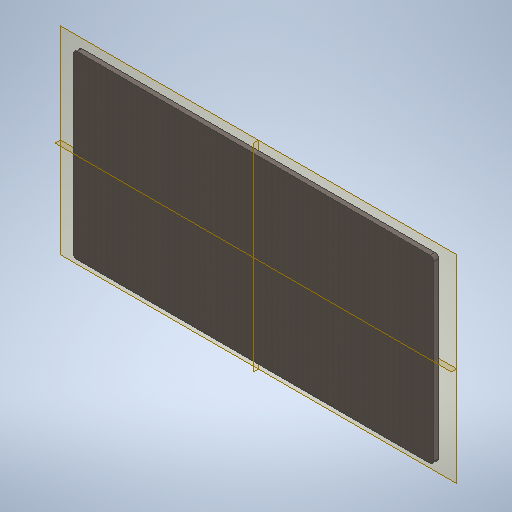
# Autodesk Inventor part: Mesa_001_0001
Saved by Autodesk Inventor 2025.2 (Build 292293000, 293)
## iProperties
Created: 2025-03-28
Part Number: Mesa_001_0001
Material: Generic
Document SubType Name: Modeling
Designer: ishad
Density: 1 g/cm^3
Appearance: Default
Author: ishad
Autodesk Inventor part; units mm, degrees
sketch "Sketch2" plane through (0, 0, 0) normal (0, 0, 1) x (1, 0, 0)
  line L0 (750, -375) -> (-750, -375)
  line L1 (-750, -375) -> (-750, 375)
  line L2 (-750, 375) -> (750, 375)
  line L3 (750, 375) -> (750, -375)
  line L4 (750, -375) -> (-750, 375) construction
  line L5 (-750, -375) -> (750, 375) construction
  point P0 (0, 0)
  dimension "d0" = 1500
  dimension "d1" = 750
  constraints: 12 end point, 2 midpoint, 2 parallel, 1 horizontal, 1 perpendicular
  measures "d0" distance of L1.end L2.end
  measures "d1" distance between parallel lines of L0 L2
extrude "Extrusion1" add sketch "Sketch2" along normal blind 20
fillet "Fillet1" radius 15 1 edges at (-750, 375, 10)
fillet "Fillet2" radius 15 1 edges at (750, 375, 10)
fillet "Fillet3" radius 15 1 edges at (750, -375, 10)
fillet "Fillet4" radius 15 1 edges at (-750, -375, 10)
body "Solid1"
